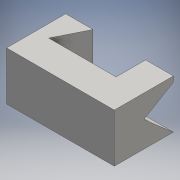
# Autodesk Inventor part: 240503_3Dsketch09
Saved by Autodesk Inventor 2016 (Build 200138000, 138)
## iProperties
Created: 2024-05-03
Part Number: 240503_3Dsketch09
Material: 일반
Document SubType Name: Modeling
Designer: pc
Density: 1 g/cm^3
Appearance: 기본값
Author: pc
Autodesk Inventor part; units mm, degrees
ref_plane "YZ Plane" through (0, 0, 0) normal (1, 0, 0) x (0, 1, 0)
ref_plane "XZ Plane" through (0, 0, 0) normal (0, 1, 0) x (-1, 0, 0)
ref_plane "XY Plane" through (0, 0, 0) normal (0, 0, 1) x (1, 0, 0)
sketch "스케치1" plane through (0, 0, 0) normal (0, 0, 1) x (1, 0, 0)
  line L0 (16.6105, -9.1135) -> (-16.6105, -9.1135)
  line L1 (-16.6105, -9.1135) -> (-16.6105, 9.1135)
  line L2 (-16.6105, 9.1135) -> (16.6105, 9.1135)
  line L3 (16.6105, 9.1135) -> (16.6105, -9.1135)
  line L4 (16.6105, -9.1135) -> (-16.6105, 9.1135) construction
  line L5 (-16.6105, -9.1135) -> (16.6105, 9.1135) construction
  point P0 (0, 0)
  constraints: 12 end point, 2 midpoint, 2 parallel, 1 horizontal, 1 perpendicular
extrude "돌출1" add sketch "스케치1" along normal blind 15
sketch "스케치2" plane through (0, 0, 15) normal (0, 0, 1) x (1, 0, 0)
  line L0 (16.6105, 9.1135) -> (-16.6105, 9.1135) projected
  line L1 (-8.2042, 9.1135) -> (-12.7307, 0)
  line L2 (-12.7307, 0) -> (8.0426, 0)
  line L3 (8.0426, 0) -> (8.0426, 9.1135)
  point P0 (0, 0)
  constraints: 6 end point, 2 point on line, 1 parallel, 1 perpendicular
extrude "돌출2" cut sketch "스케치2" against normal blind 15
sketch "스케치3" plane through (16.6105, -9.1135, 0) normal (1, 0, 0) x (0, 0, -1)
  line L0 (0, 18.2271) -> (-15, 18.2271) projected
  line L1 (-13.2965, 18.2271) -> (-7.9213, 9.1135)
  line L2 (-15, 9.1135) -> (0, 9.1135) projected
  line L3 (-7.9213, 9.1135) -> (0, 18.2271)
  constraints: 4 end point, 2 point on line
extrude "돌출3" cut sketch "스케치3" against normal blind 15
